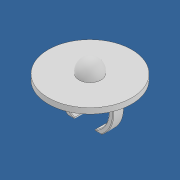
# Autodesk Inventor part: 膛轉子球座
Saved by Autodesk Inventor 2022.5 (Build 265521000, 521)
## iProperties
Created: 2024-01-31
Part Number: 膛轉子球座
Material: 一般
Document SubType Name: Modeling
Designer: 00000S04
Density: 1 g/cm^3
Appearance: 預設
Author: 普彥嘉
Autodesk Inventor part; units mm, degrees
ref_plane "YZ Plane" through (0, 0, 0) normal (1, 0, 0) x (0, 1, 0)
ref_plane "XZ Plane" through (0, 0, 0) normal (0, 1, 0) x (-1, 0, 0)
ref_plane "XY Plane" through (0, 0, 0) normal (0, 0, 1) x (1, 0, 0)
sketch "草圖1" plane through (0, 0, 0) normal (0, 0, 1) x (1, 0, 0)
  line L0 (-26.6, 0) -> (26.6, 0) construction
  line L1 (0, -6.8325) -> (0, 9.4947) construction
  line L2 (-19, 0) -> (19, 0)
  line L3 (19, 0) -> (19, -2.5)
  line L4 (19, -2.5) -> (-19, -2.5)
  line L5 (-19, -2.5) -> (-19, 0)
  circle A0 centre (0, 1) radius 5.125 construction
  arc A1 (0, 6.125) -> (-5.0265, 0) centre (0, 1) ccw
  line L6 (0, 6.125) -> (0, 0)
  line L7 (0, 0) -> (0, -2.5)
  line L8 (-19, -2.5) -> (-13.505, -4.5)
  line L9 (-13.505, -4.5) -> (0, -4.5)
  line L10 (0, -2.5) -> (0, -4.5)
  point P0 (0, 0)
  dimension "滑盤深" = 2.5
  dimension "d1" = 38
  dimension "盤球心深度" = 1
  dimension "d3" = 10.25
  dimension "盤頂拔角" = 20
  dimension "盤頂深" = 2
  constraints: 18 end point, 4 point on circle, 4 point on line, 2 centre point, 2 horizontal, 2 midpoint, 2 parallel, 1 coincident, 1 collinear, 1 concentric, 1 perpendicular, 1 vertical, 1 other
  measures "滑盤深" distance of L4.end L2.start
  measures "d1" distance of L3.end L4.end
  measures "盤球心深度" distance from line of L2 A0.centre
  measures "d3" diameter of A0
  measures "盤頂拔角" angle of L4 L8
  measures "盤頂深" distance between parallel lines of L4 L9
revolve "迴轉1" add sketch "草圖1" angle 360 about axis through (0, -10, 0) along (0, 1, 0) contours L2 L7 L4 L5 | A1 L6 L2 | L4 L10 L9 L8
sketch "草圖2" plane through (0, 0, 0) normal (0, 0, 1) x (1, 0, 0)
  line L0 (-20.6048, 0) -> (20.6048, 0) construction
  line L1 (0, -25.1175) -> (0, 7.1029) construction
  circle A0 centre (0, -8.5) radius 11 construction
  line L2 (13.505, -4.5) -> (-13.505, -4.5) construction
  arc A1 (-10.247, -4.5) -> (-3.2787, -19) centre (0, -8.5) ccw
  arc A2 (3.2787, -19) -> (10.247, -4.5) centre (0, -8.5) ccw
  arc A3 (-12.3693, -4.5) -> (-7.6649, -19) centre (0, -8.5) ccw
  arc A4 (7.6649, -19) -> (12.3693, -4.5) centre (0, -8.5) ccw
  line L3 (-7.6649, -19) -> (-3.2787, -19)
  line L4 (3.2787, -19) -> (7.6649, -19)
  line L5 (-12.3693, -4.5) -> (-10.247, -4.5)
  line L6 (10.247, -4.5) -> (12.3693, -4.5)
  point P0 (0, 0)
  dimension "d7" = 22
  dimension "拇指厚度" = 15
  dimension "d9" = 2
  dimension "拇指環至盤頂" = 14.5
  constraints: 9 point on circle, 8 end point, 5 point on line, 4 centre point, 4 horizontal, 2 coincident, 2 horizontal alignment, 1 symmetric about line, 5 other
  measures "拇指環至盤頂" distance between parallel lines of L2 L3
extrude "擠出1" add sketch "草圖2" along normal mid plane 5
fillet "圓角1" radius 0.3 12 edges at (-3.2787, -19, 0) (3.2787, -19, 0) (7.6649, -19, 0) (-7.6649, -19, 0) (-9.9146, -13.2646, 2.5) (-12.3655, -12.5119, 2.5) (-9.9146, -13.2646, -2.5) (9.9146, -13.2646, 2.5) (12.3655, -12.5119, 2.5) (-12.3655, -12.5119, -2.5) (12.3655, -12.5119, -2.5) (9.9146, -13.2646, -2.5)
fillet "圓角2" radius 0.3 20 edges at (4.7013, -18.9526, 2.5) (6.0037, -19, 2.5) (7.3775, -19, 2.4691) (7.6608, -18.9848, 2.2928) (4.5822, -18.5946, 2.4102) (4.7013, -18.9526, -2.5) (6.0037, -19, -2.5) (7.3775, -19, -2.4691) (7.6608, -18.9848, -2.2928) (4.5822, -18.5946, -2.4102) (-4.7013, -18.9526, -2.5) (-6.0037, -19, -2.5) (-7.3775, -19, -2.4691) (-7.6608, -18.9848, -2.2928) (-4.5822, -18.5946, -2.4102) (-4.7013, -18.9526, 2.5) (-6.0037, -19, 2.5) (-7.3775, -19, 2.4691) (-7.6608, -18.9848, 2.2928) (-4.5822, -18.5946, 2.4102)
equation "\"d1\" = 滑盤徑"
equation "\"盤球心深度\" = 球軸孔球心深度"
equation "\"d3\" = 球軸孔直徑"
equation "\"d7\" = 拇指環內徑"
equation "\"d9\" = 拇指環厚度"
equation "\"柱徑\" = 16"
equation "\"柱推拔角\" = 0"
equation "\"頭邊寬\" = 15"
equation "\"齒深\" = 1"
equation "\"齒邊角\" = 45deg"
equation "\"齒弧徑\" = 0.5 * 柱徑"
equation "\"齒外邊\" = 2.5"
equation "\"螺旋圈數\" = 1.5"
equation "\"螺旋推拔角\" = 0"
equation "\"d18\" = 3.488"
equation "\"d20\" = 360deg"
equation "\"孔深\" = 柱長 - 頭邊寬"
equation "\"盤深\" = 7.5"
equation "\"盤推拔角\" = 30deg"
equation "\"球軸孔直徑\" = 10.25"
equation "\"球軸孔球心深度\" = 1"
equation "\"六角孔切徑\" = 7.75"
equation "\"六角孔推拔角\" = 0"
equation "\"盤圓角\" = 0.5"
equation "\"拇指環內徑\" = 22"
equation "\"拇指環厚度\" = 2"
equation "\"滑盤徑\" = 38"
equation "\"柱長\" = 50"
